Cap for 4 inch Perforated Drain (Autodesk Fusion 360 design; units mm, degrees)
Autodesk Fusion 360 part; units mm, degrees
note: some values were not read from the file. Set by a fixed rule: which sketch regions a step uses.
sketch "Sketch3" plane through (0, 0, 0) normal (1, 0, 0) x (0, 1, 0)
  line L0 (66.675, 5) -> (57.15, 5)
  line L1 (57.15, 35) -> (52.15, 35)
  line L2 (52.15, 35) -> (52.15, 5)
  line L3 (52.15, 5) -> (0, 5)
  line L4 (57.15, 13.4069) -> (60.325, 15.24)
  line L5 (60.325, 15.24) -> (60.325, 20.24)
  line L6 (66.675, 0) -> (66.675, 5)
  line L7 (60.325, 20.24) -> (57.15, 20.24)
  line L8 (0, 0) -> (66.675, 0)
  line L9 (57.15, 5) -> (57.15, 13.4069)
  line L10 (57.15, 20.24) -> (57.15, 35)
  line L11 (0, 0) -> (0, 5)
  dimension "d9" = 5
  dimension "d11" = 5
  dimension "d14" = 5
  dimension "d15" = 30
  dimension "d16" = 57.15
  dimension "d17" = 60
  dimension "d18" = 15.24
  dimension "d19" = 60.325
  dimension "d20" = 66.675
  constraint perpendicular L0 L2
  constraint perpendicular L2 L3
  constraint perpendicular L0 L6
  constraint perpendicular L1 L9
  constraint vertical L9
  constraint vertical L5
  constraint coincident L7.end L9
  constraint perpendicular L7 L9
  constraint coincident L8.start L11.start
  constraint horizontal L3
  constraint collinear L9 L10
  constraint collinear L0 L3
  constraint coincident L6.start L8.end
  constraint horizontal L8
  constraint perpendicular L3 L11
  measures "d9" distance of L0.start L6.start
  measures "d11" distance of L4.end L5.end
  measures "d14" distance of L1.start L1.end
  measures "d15" distance of L0.end L1.start
  measures "d16" distance of L8.start L9
  measures "d17" angle of L4 L9
  measures "d18" vertical distance of L0.start L5.end
  measures "d19" horizontal distance of L8.start L5.end
  measures "d20" distance of L8.start L6.start
revolve "Revolve1" add sketch "Sketch3" angle 360 about axis through (0, 0, 1.75) along (0, 0, 1) makes body 1
sketch "Sketch4" plane through (0, 0, 5) normal (0, 0, 1) x (-1, 0, 0)
  circle A0 centre (0, 0) radius 52.15
  line L0 (-3.175, -9.525) -> (-3.175, -85.725)
  arc A1 (-3.175, -85.725) -> (3.175, -85.725) centre (0, -85.725) ccw
  line L1 (3.175, -85.725) -> (3.175, -9.525)
  arc A2 (3.175, -9.525) -> (-3.175, -9.525) centre (0, -9.525) ccw
  line L2 (0, -9.525) -> (0, -85.725) construction
  line L3 (0, -1.75) -> (0, -22.5)
  dimension "d22" = 76.2
  dimension "d23" = 6.35
  dimension "d24" = 6.35
  constraint tangent L0 A1
  constraint tangent A1 L1
  constraint parallel L0 L1
  constraint tangent L1 A2
  constraint tangent L0 A2
  constraint vertical L2
  constraint collinear L2 L3
  measures "d22" distance of A2.centre A1.centre
  measures "d23" distance of L0 L1
  measures "d24" distance of A0.centre A2
split "Split1" by face at (2.5995, 52.0852, 25) of body 1 bodies 1 makes body 2 at (-13.7168, -17.5664, 0)
extrude "Extrude3" cut sketch "Sketch4" against normal blind 5.0038 contours A0 L0 L1 A2 picked at (-0.353, -23.7297) bodies 2
pattern_linear "R-Pattern1" count 9 spacing 12.7 along (1, 0, 0) both ways of "Extrude3"
mirror "Mirror1" about plane through (0, 0, 0) normal (0, 1, 0) of "Extrude3", "R-Pattern1"
combine "Combine1" operation add target body 1 tool bodies 2
chamfer "Chamfer1" distance 2.54 angle 45 1 edges at (-53.2825, 20.6663, 35) on bodies 1
sketch "Sketch5" plane through (0, 0, 5) normal (0, 0, 1) x (-1, 0, 0)
  arc A0 (-51.7441, 6.4936) -> (-47.625, 9.525) centre (-50.8, 9.525) ccw
  arc A1 (-51.7441, 6.4936) -> (-51.7441, -6.4936) centre (0, 0) ccw
  arc A2 (-47.625, -9.525) -> (-51.7441, -6.4936) centre (-50.8, -9.525) ccw
  line L0 (-47.625, -9.525) -> (-47.625, -21.2481)
  arc A3 (-47.625, -21.2481) -> (-41.275, -31.8747) centre (0, 0) ccw
  line L1 (-41.275, -31.8747) -> (-41.275, -9.525)
  arc A4 (-34.925, -9.525) -> (-41.275, -9.525) centre (-38.1, -9.525) ccw
  line L2 (-34.925, -9.525) -> (-34.925, -38.7281)
  arc A5 (-34.925, -38.7281) -> (-28.575, -43.6244) centre (0, 0) ccw
  line L3 (-28.575, -43.6244) -> (-28.575, -9.525)
  arc A6 (-22.225, -9.525) -> (-28.575, -9.525) centre (-25.4, -9.525) ccw
  line L4 (-22.225, -9.525) -> (-22.225, -47.177)
  arc A7 (-22.225, -47.177) -> (-15.875, -49.675) centre (0, 0) ccw
  line L5 (-15.875, -49.675) -> (-15.875, -9.525)
  arc A8 (-9.525, -9.525) -> (-15.875, -9.525) centre (-12.7, -9.525) ccw
  line L6 (-9.525, -9.525) -> (-9.525, -51.2728)
  arc A9 (-9.525, -51.2728) -> (-3.175, -52.0533) centre (0, 0) ccw
  line L7 (-3.175, -52.0533) -> (-3.175, -9.525)
  arc A10 (3.175, -9.525) -> (-3.175, -9.525) centre (0, -9.525) ccw
  line L8 (3.175, -9.525) -> (3.175, -52.0533)
  arc A11 (3.175, -52.0533) -> (9.525, -51.2728) centre (0, 0) ccw
  line L9 (9.525, -51.2728) -> (9.525, -9.525)
  arc A12 (15.875, -9.525) -> (9.525, -9.525) centre (12.7, -9.525) ccw
  line L10 (15.875, -9.525) -> (15.875, -49.675)
  arc A13 (15.875, -49.675) -> (22.225, -47.177) centre (0, 0) ccw
  line L11 (22.225, -47.177) -> (22.225, -9.525)
  arc A14 (28.575, -9.525) -> (22.225, -9.525) centre (25.4, -9.525) ccw
  line L12 (28.575, -9.525) -> (28.575, -43.6244)
  arc A15 (28.575, -43.6244) -> (34.925, -38.7281) centre (0, 0) ccw
  line L13 (34.925, -38.7281) -> (34.925, -9.525)
  arc A16 (41.275, -9.525) -> (34.925, -9.525) centre (38.1, -9.525) ccw
  line L14 (41.275, -9.525) -> (41.275, -31.8747)
  arc A17 (41.275, -31.8747) -> (47.625, -21.2481) centre (0, 0) ccw
  line L15 (47.625, -21.2481) -> (47.625, -9.525)
  arc A18 (51.7441, -6.4936) -> (47.625, -9.525) centre (50.8, -9.525) ccw
  arc A19 (51.7441, -6.4936) -> (51.7441, 6.4936) centre (0, 0) ccw
  arc A20 (47.625, 9.525) -> (51.7441, 6.4936) centre (50.8, 9.525) ccw
  line L16 (47.625, 9.525) -> (47.625, 21.2481)
  arc A21 (47.625, 21.2481) -> (41.275, 31.8747) centre (0, 0) ccw
  line L17 (41.275, 31.8747) -> (41.275, 9.525)
  arc A22 (34.925, 9.525) -> (41.275, 9.525) centre (38.1, 9.525) ccw
  line L18 (34.925, 9.525) -> (34.925, 38.7281)
  arc A23 (34.925, 38.7281) -> (28.575, 43.6244) centre (0, 0) ccw
  line L19 (28.575, 43.6244) -> (28.575, 9.525)
  arc A24 (22.225, 9.525) -> (28.575, 9.525) centre (25.4, 9.525) ccw
  line L20 (22.225, 9.525) -> (22.225, 47.177)
  arc A25 (22.225, 47.177) -> (15.875, 49.675) centre (0, 0) ccw
  line L21 (15.875, 49.675) -> (15.875, 9.525)
  arc A26 (9.525, 9.525) -> (15.875, 9.525) centre (12.7, 9.525) ccw
  line L22 (9.525, 9.525) -> (9.525, 51.2728)
  arc A27 (9.525, 51.2728) -> (3.175, 52.0533) centre (0, 0) ccw
  line L23 (3.175, 52.0533) -> (3.175, 9.525)
  arc A28 (-3.175, 9.525) -> (3.175, 9.525) centre (0, 9.525) ccw
  line L24 (-3.175, 9.525) -> (-3.175, 52.0533)
  arc A29 (-3.175, 52.0533) -> (-9.525, 51.2728) centre (0, 0) ccw
  line L25 (-9.525, 51.2728) -> (-9.525, 9.525)
  arc A30 (-15.875, 9.525) -> (-9.525, 9.525) centre (-12.7, 9.525) ccw
  line L26 (-15.875, 9.525) -> (-15.875, 49.675)
  arc A31 (-15.875, 49.675) -> (-22.225, 47.177) centre (0, 0) ccw
  line L27 (-22.225, 47.177) -> (-22.225, 9.525)
  arc A32 (-28.575, 9.525) -> (-22.225, 9.525) centre (-25.4, 9.525) ccw
  line L28 (-28.575, 9.525) -> (-28.575, 43.6244)
  arc A33 (-28.575, 43.6244) -> (-34.925, 38.7281) centre (0, 0) ccw
  line L29 (-34.925, 38.7281) -> (-34.925, 9.525)
  arc A34 (-41.275, 9.525) -> (-34.925, 9.525) centre (-38.1, 9.525) ccw
  line L30 (-41.275, 9.525) -> (-41.275, 31.8747)
  arc A35 (-41.275, 31.8747) -> (-47.625, 21.2481) centre (0, 0) ccw
  line L31 (-47.625, 21.2481) -> (-47.625, 9.525)
  line L32 (52.0533, 3.175) -> (-52.0533, 3.175)
  line L33 (-20, 0) -> (-2.5, 0)
  line L34 (52.0533, -3.175) -> (-52.0533, -3.175)
  dimension "d34" = 6.35
  constraint coincident A19 L32.start
  constraint coincident A1 L32.end
  constraint horizontal L32
  constraint symmetric L32.start L33 L34.start
  constraint symmetric L32.end L33 L34.end
  measures "d34" distance of L32 L34
extrude "Extrude4" add sketch "Sketch5" along normal blind 6.35 contours A1 A19 L32 L34 bodies 1
move_body "Move1" bodies 1 to x (1, 0, 0) y (0, -1, 0) z (0, 0, -1) at (0, -133.35, 0)
equation "d16 = ( 4.5 / 2 ) * 1 in"
equation "d19 = ( 4.75 / 2 ) * 1 in"
equation "d20 = ( 5.25 / 2 ) * 1 in"
